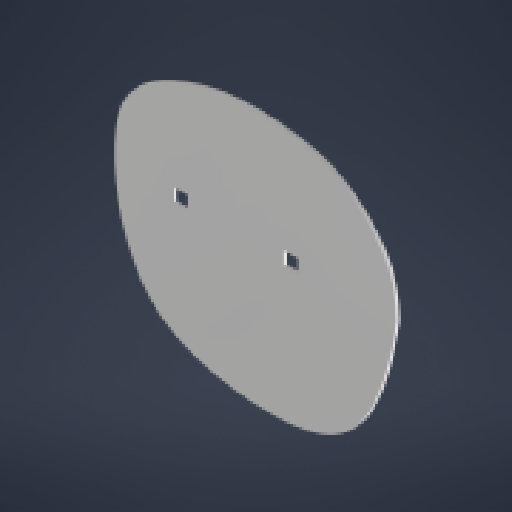
# Autodesk Inventor part: hori-side
Saved by Autodesk Inventor 2023.2 (Build 272271000, 271)
## iProperties
Created: 2023-04-15
Part Number: hori-side
Material: Polycarbonate, Clear
Document SubType Name: Modeling
Designer: Liam
Density: 1.2 g/cm^3
Appearance: Polycarbonate - Clear
Author: Liam
Autodesk Inventor part; units mm, degrees
ref_plane "YZ Plane" through (0, 0, 0) normal (1, 0, 0) x (0, 1, 0)
ref_plane "XZ Plane" through (0, 0, 0) normal (0, 1, 0) x (-1, 0, 0)
ref_plane "XY Plane" through (0, 0, 0) normal (0, 0, 1) x (1, 0, 0)
sketch "Sketch1" plane through (0, 0, 0) normal (0, 0, 1) x (1, 0, 0)
  arc A0 (2.555, -3.19) -> (3.19, -2.555) centre (2.555, -2.555) ccw projected
  line L0 (3.19, -2.555) -> (3.19, 2.555) projected
  arc A1 (3.19, 2.555) -> (2.555, 3.19) centre (2.555, 2.555) ccw projected
  line L1 (2.555, 3.19) -> (-2.555, 3.19) projected
  arc A2 (-2.555, 3.19) -> (-3.19, 2.555) centre (-2.555, 2.555) ccw projected
  line L2 (-3.19, 2.555) -> (-3.19, -2.555) projected
  arc A3 (-3.19, -2.555) -> (-2.555, -3.19) centre (-2.555, -2.555) ccw projected
  line L3 (-2.555, -3.19) -> (2.555, -3.19) projected
  arc A4 (-53.99, -2.555) -> (-53.355, -3.19) centre (-53.355, -2.555) ccw
  line L4 (-53.355, -3.19) -> (-48.245, -3.19)
  arc A5 (-48.245, -3.19) -> (-47.61, -2.555) centre (-48.245, -2.555) ccw
  line L5 (-47.61, -2.555) -> (-47.61, 2.555)
  arc A6 (-47.61, 2.555) -> (-48.245, 3.19) centre (-48.245, 2.555) ccw
  line L6 (-48.245, 3.19) -> (-53.355, 3.19)
  arc A7 (-53.355, 3.19) -> (-53.99, 2.555) centre (-53.355, 2.555) ccw
  line L7 (-53.99, 2.555) -> (-53.99, -2.555)
  line L8 (-50.8, 0) -> (-53.99, 0) construction
  line L9 (-50.8, 0) -> (-50.8, -3.19) construction
  line L10 (-50.8, 0) -> (-47.61, 0) construction
  line L11 (-50.8, 0) -> (-50.8, 3.19) construction
  line L12 (48.6294, 0) -> (43.7245, -28.5469) construction
  line L13 (43.7245, -28.5469) -> (31.7563, -55.0338) construction
  line L14 (31.7563, -55.0338) -> (12.5288, -64.2552) construction
  line L15 (12.5288, -64.2552) -> (-14.5466, -66.2172) construction
  line L16 (-14.5466, -66.2172) -> (-46.3309, -61.116) construction
  line L17 (-46.3309, -61.116) -> (-70.2671, -47.1859) construction
  line L18 (-70.2671, -47.1859) -> (-82.2353, -12.851) construction
  line L19 (-82.2353, -12.851) -> (-82.2353, 18.5408) construction
  line L20 (-82.2353, 18.5408) -> (-72.4253, 37.7683) construction
  line L21 (-72.4253, 37.7683) -> (-43.7803, 49.9326) construction
  line L22 (-43.7803, 49.9326) -> (-20.4326, 53.8566) construction
  line L23 (-20.4326, 53.8566) -> (8.9972, 50.5212) construction
  line L24 (8.9972, 50.5212) -> (23.9084, 45.2239) construction
  line L25 (23.9084, 45.2239) -> (40.3891, 30.3127) construction
  line L26 (40.3891, 30.3127) -> (46.8636, 18.5408) construction
  line L27 (46.8636, 18.5408) -> (48.6294, 7.1613) construction
  line L28 (48.6294, 7.1613) -> (48.6294, 0) construction
  spline S0 degree 4 poles (48.6294, 0) (43.7245, -28.5469) (31.7563, -55.0338) (12.5288, -64.2552) (-14.5466, -66.2172) (-46.3309, -61.116) (-70.2671, -47.1859) (-82.2353, -12.851) (-82.2353, 18.5408) (-72.4253, 37.7683) (-43.7803, 49.9326) (-20.4326, 53.8566) (8.9972, 50.5212) (23.9084, 45.2239) (40.3891, 30.3127) (46.8636, 18.5408) (48.6294, 7.1613) (48.6294, 0) knots 1 1 1 1 1 2 3 4 5 6 7 8 9 10 11 12 13 14 15 15 15 15 15
  point P0 (0, 0)
  dimension "d0" = 6.38
  dimension "d1" = 6.38
  dimension "d3" = 0.635
  dimension "d4" = 0
  dimension "d5" = 50.8
  constraints: 16 end point, 8 point on circle, 5 equal length, 5 tangent, 4 centre point, 4 midpoint, 3 equal radius, 3 perpendicular, 2 point on line, 2 vertical, 1 parallel, 2 other
  measures "d0" distance between parallel lines of L6 L4
  measures "d1" distance between parallel lines of L7 L5
  measures "d3" radius of A5
  measures "d4" vertical distance of point (0, 0) L8.start
  measures "d5" distance of point (0, 0) L8.start
extrude "Extrusion1" add sketch "Sketch1" along normal blind 1.524
equation "\"d1\" = d0"
body "Solid1"
